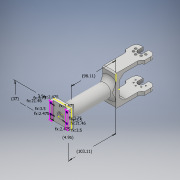
# Autodesk Inventor part: HuesitoJustina2
Saved by Autodesk Inventor 2018 (Build 220112000, 112)
## iProperties
Created: 2019-04-23
Part Number: HuesitoJustina2
Material: Genérico
Document SubType Name: Modeling
Designer: kille
Density: 1 g/cm^3
Appearance: Valor por defecto
Author: kille
Autodesk Inventor part; units mm, degrees
ref_plane "YZ Plane" through (0, 0, 0) normal (1, 0, 0) x (0, 1, 0)
ref_plane "XZ Plane" through (0, 0, 0) normal (0, 1, 0) x (-1, 0, 0)
ref_plane "XY Plane" through (0, 0, 0) normal (0, 0, 1) x (1, 0, 0)
sketch "Boceto1" plane through (0, 0, 0) normal (0, 1, 0) x (-1, 0, 0)
  line L0 (14.5, 26) -> (-14.5, 26)
  line L1 (-14.5, 26) -> (-14.5, -26)
  line L2 (-14.5, -26) -> (14.5, -26)
  line L3 (14.5, -26) -> (14.5, 26)
  point P0 (0, 0)
  dimension "d0" = 52
  dimension "d1" = 29
  dimension "d2" = 14.5
  dimension "d3" = 26
  constraints: 8 end point, 2 parallel, 1 horizontal, 1 perpendicular
  measures "d0" distance of L2.end L0.start
  measures "d1" distance of L0.start L0.end
  measures "d2" distance from line of point (0, 0) L3
  measures "d3" distance from line of point (0, 0) L0
extrude "Extrusión1" add sketch "Boceto1" against normal blind 7.5
sketch "Boceto2" plane through (-14.5, 0, 26) normal (0, 0, 1) x (1, 0, 0)
  line L0 (0, 0) -> (29, 0) projected
  line L1 (0, 0) -> (29, 0) projected
  line L2 (0, 0) -> (0, -7.5) projected
  line L3 (29, -7.5) -> (0, -7.5) projected
  line L4 (29, 0) -> (29, -7.5) projected
  line L5 (0, 0) -> (29, 0)
  line L6 (29, 0) -> (29, 67)
  line L7 (29, 67) -> (0, 67)
  line L8 (0, 67) -> (0, 0)
  point P0 (14.5, 0)
  dimension "d6" = 29
  dimension "d7" = 67
  dimension "d8" = 29
  constraints: 8 end point, 2 parallel, 1 horizontal, 1 perpendicular
  measures "d6" distance of L3.start L2.end
  measures "d7" distance of L5.end L6.end
  measures "d8" distance of L6.end L7.end
extrude "Extrusión2" add sketch "Boceto2" along normal blind 7.5 contours L8 L7 L6 L0
sketch "Boceto3" plane through (14.5, 0, -26) normal (0, 0, -1) x (-1, 0, 0)
  line L0 (29, 0) -> (0, 0) projected
  line L1 (29, 67) -> (29, 0) projected
  line L2 (0, 67) -> (29, 67) projected
  line L3 (0, 0) -> (0, 67) projected
  line L4 (0, 0) -> (29, 0) projected
  line L5 (0, 0) -> (0, -7.5) projected
  line L6 (29, -7.5) -> (0, -7.5) projected
  line L7 (29, 0) -> (29, -7.5) projected
  point P0 (14.5, 0)
extrude "Extrusión3" add sketch "Boceto3" along normal blind 7.5 contours L0 L3 L2 L1
sketch "Boceto4" plane through (14.5, -7.5, 26) normal (1, 0, 0) x (0, 0, -1)
  line L0 (52, 7.5) -> (52, 0) projected
  line L1 (52, 7.5) -> (59.5, 7.5) projected
  line L2 (0, 7.5) -> (-7.5, 7.5) projected
  line L3 (0, 7.5) -> (0, 0) projected
  line L4 (0, 7.5) -> (-7.5, 7.5)
  line L5 (-7.5, 7.5) -> (-7.5, 0)
  line L6 (-7.5, 0) -> (0, 0)
  line L7 (0, 0) -> (0, 7.5)
  line L8 (52, 7.5) -> (59.5, 7.5)
  line L9 (59.5, 7.5) -> (59.5, 0)
  line L10 (59.5, 0) -> (52, 0)
  line L11 (52, 0) -> (52, 7.5)
  point P0 (26, 7.5)
  dimension "d13" = 7.5
  dimension "d14" = 7.5
  dimension "d15" = 7.5
  dimension "d16" = 7.5
  constraints: 16 end point, 4 parallel, 2 horizontal, 2 perpendicular, 1 point on line
  measures "d13" distance of L8.end L9.end
  measures "d14" distance of L9.end L10.end
  measures "d15" distance of L4.end L5.end
  measures "d16" distance of L5.end L6.end
extrude "Extrusión4" add sketch "Boceto4" against normal blind 29
sketch "Boceto5" plane through (14.5, 0, 26) normal (1, 0, 0) x (0, 0, -1)
  line L0 (0, 0) -> (0, 67) projected
  line L1 (0, 0) -> (52, 0) projected
  line L2 (52, 67) -> (52, 0) projected
  line L3 (52, 0) -> (0, 0) projected
  line L4 (0, 10) -> (10, 0)
  line L5 (42, 0) -> (52, 10)
  point P0 (26, 0)
  dimension "d19" = 10
  dimension "d20" = 10
  dimension "d21" = 10
  dimension "d22" = 10
  constraints: 4 end point, 4 point on line
  measures "d19" distance of L0.start L4.start
  measures "d20" distance of L0.start L4.end
  measures "d21" distance of L1.end L5.start
  measures "d22" distance of L5.end L1.end
extrude "Extrusión5" add sketch "Boceto5" against normal blind 29
sketch "Boceto6" plane through (0, -7.5, 0) normal (0, -1, 0) x (1, 0, 0)
  circle A0 centre (0, 0) radius 14
  dimension "d26" = 28
  constraints: 1 centre point, 1 coincident
  measures "d26" diameter of A0
extrude "Extrusión6" add sketch "Boceto6" along normal blind 103.11
fillet "Empalme1" radius 10 1 edges at (-14, -7.5, 0)
fillet "Empalme2" radius 10 4 edges at (0, 10, -26) (0, 0, -16) (0, 0, 16) (0, 10, 26)
sketch "Boceto7" plane through (14.5, 0, -33.5) normal (0, 0, -1) x (-1, 0, 0)
  line L0 (29, 67) -> (29, -7.5) projected
  line L1 (29, 67) -> (0, 67) projected
  line L2 (0, 67) -> (0, -7.5) projected
  line L3 (0, -7.5) -> (29, -7.5) projected
  line L4 (29, 67) -> (0, 67) projected
  line L5 (19.5, 67) -> (9.5, 67)
  line L6 (9.5, 67) -> (9.5, 62)
  line L7 (9.5, 62) -> (19.5, 62)
  line L8 (19.5, 62) -> (19.5, 67)
  arc A0 (9.5, 62) -> (19.5, 62) centre (14.5, 62) ccw
  circle A1 centre (14.5, 50.85) radius 1.35
  circle A2 centre (25.65, 62) radius 1.35
  circle A3 centre (3.35, 62) radius 1.35
  circle A4 centre (22.6295, 54.3689) radius 1.35
  circle A5 centre (6.1262, 54.6378) radius 1.35
  point P0 (14.5, 0)
  point P1 (14.5, 67)
  dimension "d31" = 29
  dimension "d32" = 74.5
  dimension "d33" = 14.5
  dimension "d34" = 10
  dimension "d35" = 5
  dimension "d36" = 5
  dimension "d37" = 5
  dimension "d38" = 2.7
  dimension "d39" = 4.8
  dimension "d40" = 2.7
  dimension "d41" = 2.7
  dimension "d43" = 11.15
  dimension "d44" = 11.15
  dimension "d45" = 11.15
  dimension "d46" = 2.7
  dimension "d47" = 2.7
  dimension "d48" = 11.15
  dimension "d49" = 11.15
  constraints: 8 end point, 6 centre point, 2 parallel, 2 point on circle, 1 horizontal, 1 midpoint, 1 perpendicular, 1 point on line
  measures "d31" distance of L0.start L1.end
  measures "d32" distance of L0.start L0.end
  measures "d33" distance of point (14.5, 67) L0.start
  measures "d34" distance of L6.end L7.end
  measures "d35" distance of point (14.5, 67) L5.start
  measures "d36" distance of L7.end L5.start
  measures "d37" radius of A0
  measures "d38" diameter of A1
  measures "d40" diameter of A2
  measures "d41" diameter of A3
  measures "d43" distance of A1.centre A0.centre
  measures "d44" distance of A2.centre A0.centre
  measures "d45" distance of A0.centre A3.centre
  measures "d46" diameter of A4
  measures "d47" diameter of A5
  measures "d48" distance of A4.centre A0.centre
  measures "d49" distance of A5.centre A0.centre
extrude "Extrusión7" cut sketch "Boceto7" against normal blind 67 contours L8 L7 L6 L1 | A0 L7 | A1 | A2 | A3 | A4 | A5
sketch "Boceto8" plane through (0, -110.61, 0) normal (0, -1, 0) x (1, 0, 0)
  circle A0 centre (0, 0) radius 14 projected
  line L0 (20.125, 21.1) -> (-20.125, 21.1)
  line L1 (-20.125, 21.1) -> (-20.125, -19.15)
  line L2 (-20.125, -19.15) -> (20.125, -19.15)
  line L3 (20.125, -19.15) -> (20.125, 21.1)
  dimension "d52" = 40.25
  dimension "d53" = 40.25
  dimension "d55" = 28
  dimension "d89" = 20.125
  dimension "d90" = 21.1
  constraints: 8 end point, 2 parallel, 1 horizontal, 1 perpendicular
  measures "d52" distance of L2.end L0.start
  measures "d53" distance of L0.start L0.end
  measures "d55" diameter of A0
  measures "d89" distance from line of point (0, 0) L1
  measures "d90" distance from line of L0 point (0, 0)
extrude "Extrusión8" add sketch "Boceto8" along normal blind 4 contours A0 | L3 L2 L1 L0
sketch "Boceto14" plane through (-14.5, 0, 33.5) normal (0, 0, 1) x (1, 0, 0)
  circle A0 centre (3.35, 62) radius 1.35 projected
  circle A1 centre (6.3705, 54.3689) radius 1.35 projected
  circle A2 centre (14.5, 50.85) radius 1.35 projected
  circle A3 centre (22.8738, 54.6378) radius 1.35 projected
  circle A4 centre (25.65, 62) radius 1.35 projected
  circle A5 centre (3.35, 62) radius 2.4
  circle A6 centre (6.3705, 54.3689) radius 2.4
  circle A7 centre (14.5, 50.85) radius 2.4
  circle A8 centre (22.8738, 54.6378) radius 2.4
  circle A9 centre (25.65, 62) radius 2.4
  point P0 (14.5, 0)
  dimension "d91" = 4.8
  dimension "d92" = 4.8
  dimension "d93" = 4.8
  dimension "d94" = 4.8
  dimension "d95" = 4.8
  constraints: 5 centre point, 5 coincident
  measures "d91" diameter of A5
  measures "d92" diameter of A6
  measures "d93" diameter of A7
  measures "d94" diameter of A8
  measures "d95" diameter of A9
extrude "Extrusión14" cut sketch "Boceto14" against normal blind 5.5 contours A0 | A1 | A2 | A3 | A4 | A5 | A6 | A7 | A8 | A9
sketch "Boceto15" plane through (14.5, 0, -33.5) normal (0, 0, -1) x (-1, 0, 0)
  circle A0 centre (25.65, 62) radius 1.35 projected
  circle A1 centre (25.65, 62) radius 2.4 projected
  circle A2 centre (22.6295, 54.3689) radius 1.35 projected
  circle A3 centre (22.6295, 54.3689) radius 2.4 projected
  circle A4 centre (14.5, 50.85) radius 1.35 projected
  circle A5 centre (14.5, 50.85) radius 2.4 projected
  circle A6 centre (6.1262, 54.6378) radius 1.35 projected
  circle A7 centre (6.1262, 54.6378) radius 2.4 projected
  circle A8 centre (3.35, 62) radius 1.35 projected
  circle A9 centre (3.35, 62) radius 2.4 projected
  point P0 (14.5, 0)
extrude "Extrusión15" cut sketch "Boceto15" against normal blind 5.5 contours A0 | A1 | A2 | A3 | A4 | A5 | A6 | A7 | A8 | A9
sketch "Boceto16" plane through (0, -114.61, 0) normal (0, -1, 0) x (1, 0, 0)
  circle A0 centre (0, 0) radius 14 projected
  circle A1 centre (0, 0) radius 6.5
  dimension "d100" = 13
  constraints: 1 centre point, 1 coincident
  measures "d100" diameter of A1
extrude "Extrusión16" cut sketch "Boceto16" against normal blind 5 contours A1
sketch "Boceto17" plane through (0, -114.61, 0) normal (0, -1, 0) x (1, 0, 0)
  circle A0 centre (0, 0) radius 6.5 projected
  line L0 (20.125, 21.1) -> (-20.125, 21.1) projected
  line L1 (-20.125, 21.1) -> (-20.125, -19.15) projected
  line L2 (-20.125, -19.15) -> (20.125, -19.15) projected
  line L3 (20.125, -19.15) -> (20.125, 21.1) projected
  line L4 (-20.125, 21.1) -> (-20.125, -19.15) projected
  line L5 (-20.125, 21.1) -> (-15.175, 21.1)
  line L6 (-15.175, 21.1) -> (-15.175, -15.9)
  line L7 (-15.175, -15.9) -> (-20.125, -15.9)
  line L8 (-20.125, -15.9) -> (-20.125, 21.1)
  line L9 (20.125, 21.1) -> (15.175, 21.1)
  line L10 (15.175, 21.1) -> (15.175, -15.9)
  line L11 (15.175, -15.9) -> (20.125, -15.9)
  line L12 (20.125, -15.9) -> (20.125, 21.1)
  dimension "d103" = 37
  dimension "d104" = 4.95
  dimension "d105" = 37
  dimension "d106" = 4.95
  constraints: 16 end point, 4 parallel, 2 horizontal, 2 perpendicular
  measures "d103" distance of L5.end L6.end
  measures "d104" distance of L6.end L7.end
  measures "d105" distance of L9.end L10.end
  measures "d106" distance of L10.end L11.end
extrude "Extrusión17" add sketch "Boceto17" along normal blind 4 contours L3 L11 L10 L0 | L6 L7 L1 L0
sketch "Boceto18" plane through (-20.125, -110.61, -19.15) normal (-1, 0, 0) x (0, 0, 1)
  line L0 (40.25, 0) -> (0, 0) projected
  line L1 (0, 0) -> (0, -4) projected
  line L2 (3.25, -4) -> (0, -4) projected
  line L3 (3.25, -4) -> (3.25, -8) projected
  line L4 (40.25, -8) -> (3.25, -8) projected
  line L5 (40.25, 0) -> (40.25, -8) projected
  line L6 (0, 0) -> (0, -4) projected
  line L7 (0, 0) -> (3.25, -8)
  line L8 (3.25, -4) -> (3.25, -8) projected
  line L9 (3.25, -8) -> (3.25, -4)
  line L10 (3.25, -4) -> (1.625, -4)
  line L11 (0, -4) -> (3.25, -4) projected
  point P0 (19.15, 110.61)
  constraints: 6 end point, 2 midpoint, 1 collinear
extrude "Extrusión18" add sketch "Boceto18" against normal blind 4.95 contours L2 L3 L7
sketch "Boceto19" plane through (-20.125, -110.61, -19.15) normal (-1, 0, 0) x (0, 0, 1)
  line L0 (40.25, 0) -> (0, 0) projected
  line L1 (0, 0) -> (0, -4) projected
  line L2 (1.625, -4) -> (0, -4) projected
  line L3 (1.625, -4) -> (3.25, -8) projected
  line L4 (40.25, -8) -> (3.25, -8) projected
  line L5 (40.25, 0) -> (40.25, -8) projected
  line L6 (0, 0) -> (1.625, -4)
  line L7 (0, -4) -> (3.25, -4) projected
  line L8 (0, 0) -> (0, -4)
  line L9 (0, -4) -> (1.625, -4)
  point P0 (19.15, 110.61)
  constraints: 6 end point, 1 collinear, 1 perpendicular
extrude "Extrusión19" cut sketch "Boceto19" against normal blind 40.5 contours L6 L2 L1
sketch "Boceto20" plane through (20.125, -118.61, 21.1) normal (1, 0, 0) x (0, 0, -1)
  line L0 (38.625, 4) -> (40.25, 8) projected
  line L1 (40.25, 8) -> (0, 8) projected
  line L2 (0, 8) -> (0, 0) projected
  line L3 (37, 0) -> (0, 0) projected
  line L4 (37, 4) -> (37, 0) projected
  line L5 (38.625, 4) -> (37, 4) projected
  line L6 (37, 0) -> (38.625, 4) projected
  point P0 (21.1, 118.61)
extrude "Extrusión20" add sketch "Boceto20" against normal blind 4.95 contours L6 L4 L5
sketch "Boceto21" plane through (0, -118.61, 0) normal (0, -1, 0) x (1, 0, 0)
  line L0 (-20.125, 21.1) -> (-20.125, -15.9) projected
  line L1 (-20.125, -15.9) -> (-15.175, -15.9) projected
  line L2 (-15.175, -15.9) -> (-15.175, 21.1) projected
  line L3 (-15.175, 21.1) -> (-20.125, 21.1) projected
  line L4 (20.125, 21.1) -> (15.175, 21.1) projected
  line L5 (15.175, 21.1) -> (15.175, -15.9) projected
  line L6 (15.175, -15.9) -> (20.125, -15.9) projected
  line L7 (20.125, -15.9) -> (20.125, 21.1) projected
  circle A0 centre (-17.65, 17.35) radius 1.75
  circle A1 centre (-17.65, -4.11) radius 1.75
  circle A2 centre (17.65, 17.35) radius 1.75
  circle A3 centre (17.65, -4.11) radius 1.75
  line L8 (-20.125, 21.1) -> (-20.125, -15.9) projected
  line L9 (-20.125, -15.9) -> (-15.175, -15.9) projected
  line L10 (-15.175, -15.9) -> (-15.175, 21.1) projected
  line L11 (-15.175, 21.1) -> (-20.125, 21.1) projected
  line L12 (20.125, 21.1) -> (15.175, 21.1) projected
  line L13 (15.175, 21.1) -> (15.175, -15.9) projected
  line L14 (20.125, -15.9) -> (20.125, 21.1) projected
  line L15 (15.175, -15.9) -> (20.125, -15.9) projected
  point P0 (0, 0)
  dimension "d115" = 3.5
  dimension "d116" = 3.75
  dimension "d117" = 3.75
  dimension "d118" = 2.475
  dimension "d119" = 2.475
  dimension "d120" = 3.5
  dimension "d121" = 3.5
  dimension "d122" = 3.5
  dimension "d123" = 21.46
  dimension "d124" = 21.46
  dimension "d125" = 2.475
  dimension "d126" = 2.475
  dimension "d129" = 4.95
  dimension "d172" = 37
  constraints: 4 centre point
  measures "d115" diameter of A0
  measures "d116" distance from line of A0.centre L3
  measures "d117" distance from line of L4 A2.centre
  measures "d118" distance from line of L0 A0.centre
  measures "d119" distance from line of L7 A2.centre
  measures "d120" diameter of A2
  measures "d121" diameter of A1
  measures "d122" diameter of A3
  measures "d123" distance of A1.centre A0.centre
  measures "d124" distance of A2.centre A3.centre
  measures "d125" distance from line of L7 A3.centre
  measures "d126" distance from line of L0 A1.centre
  measures "d129" distance of L5.end L6.end
  measures "d172" distance of L0.start L0.end
sketch "Boceto22" plane through (0, -110.61, 0) normal (0, 1, 0) x (1, 0, 0)
  line L0 (20.125, -21.1) -> (-20.125, -21.1) projected
  line L1 (20.125, 19.15) -> (20.125, -21.1) projected
  line L2 (-20.125, 19.15) -> (20.125, 19.15) projected
  line L3 (-20.125, -21.1) -> (-20.125, 19.15) projected
  circle A0 centre (0, 0) radius 14 projected
sketch "Boceto23" plane through (-14.5, 0, 33.5) normal (0, 0, 1) x (1, 0, 0)
  circle A0 centre (22.8738, 54.6378) radius 2.4 projected
  circle A1 centre (6.3705, 54.3689) radius 2.4 projected
  circle A2 centre (3.35, 62) radius 2.4 projected
  circle A3 centre (14.5, 50.85) radius 2.4 projected
  circle A4 centre (25.65, 62) radius 2.4 projected
  line L0 (19.5, 67) -> (19.5, 62) projected
  arc A5 (9.5, 62) -> (19.5, 62) centre (14.5, 62) ccw projected
  line L1 (9.5, 62) -> (9.5, 67) projected
  line L2 (9.5, 67) -> (0, 67) projected
  line L3 (0, 67) -> (0, -7.5) projected
  line L4 (29, -7.5) -> (0, -7.5) projected
  line L5 (29, 67) -> (29, -7.5) projected
  line L6 (29, 67) -> (19.5, 67) projected
  line L7 (9.5, 67) -> (9.5, 62) projected
  line L8 (9.5, 67) -> (19.5, 67)
  line L9 (19.5, 67) -> (19.5, 62)
  line L10 (19.5, 62) -> (9.5, 62)
  line L11 (9.5, 62) -> (9.5, 67)
  line L12 (0, 67) -> (9.5, 67) projected
  arc A6 (9.5, 62) -> (19.5, 62) centre (14.5, 62) ccw projected
  line L13 (6.3705, 67) -> (9.5, 67)
  line L14 (9.5, 67) -> (9.5, 62)
  line L15 (9.5, 62) -> (6.3705, 62)
  line L16 (6.3705, 62) -> (6.3705, 67)
  line L17 (19.5, 67) -> (22.6295, 67)
  line L18 (22.6295, 67) -> (22.6295, 62)
  line L19 (22.6295, 62) -> (19.5, 62)
  line L20 (19.5, 62) -> (19.5, 67)
  line L21 (7.9352, 62) -> (7.9352, 67)
  line L22 (21.0648, 62) -> (21.0648, 67)
  line L23 (7.9352, 62) -> (9.5, 62)
  line L24 (9.5, 62) -> (9.5, 67)
  line L25 (9.5, 67) -> (7.9352, 67)
  line L26 (7.9352, 67) -> (7.9352, 62)
  line L27 (19.5, 62) -> (21.0648, 62)
  line L28 (21.0648, 62) -> (21.0648, 67)
  line L29 (21.0648, 67) -> (19.5, 67)
  line L30 (19.5, 67) -> (19.5, 62)
  line L31 (6.3705, 62) -> (7.9352, 62)
  line L32 (7.9352, 62) -> (7.9352, 67)
  line L33 (7.9352, 67) -> (6.3705, 67)
  line L34 (6.3705, 67) -> (6.3705, 62)
  line L35 (22.6295, 62) -> (21.0648, 62)
  line L36 (21.0648, 62) -> (21.0648, 67)
  line L37 (21.0648, 67) -> (22.6295, 67)
  line L38 (22.6295, 67) -> (22.6295, 62)
  arc A7 (6.3705, 62) -> (22.6295, 62) centre (14.5, 62) ccw
  point P0 (14.5, 0)
  dimension "d135" = 5
  dimension "d136" = 3.1295
  dimension "d137" = 3.1295
  constraints: 60 end point, 14 parallel, 7 horizontal, 7 perpendicular, 4 midpoint, 3 point on circle, 3 point on line, 1 centre point, 1 tangent
  measures "d135" distance of L15.end L13.start
  measures "d136" distance of L14.end L15.end
  measures "d137" distance of L18.end L19.end
extrude "Extrusión23" cut sketch "Boceto23" against normal blind 67 contours L6 L22 L19 L0 | L0 L10 L1 L8 | L19 A7 L15 A5 | A5 L10 | L6 L18 L19 L22 | L1 L15 L21 L2 | L21 L15 L16 L2
sketch "Boceto24" plane through (-14.5, 0, 33.5) normal (0, 0, 1) x (1, 0, 0)
  line L0 (22.6295, 67) -> (22.6295, 62) projected
  arc A0 (6.3705, 62) -> (22.6295, 62) centre (14.5, 62) ccw projected
  line L1 (6.3705, 62) -> (6.3705, 67) projected
  line L2 (6.3705, 67) -> (0, 67) projected
  line L3 (0, 67) -> (0, -7.5) projected
  line L4 (29, -7.5) -> (0, -7.5) projected
  line L5 (29, 67) -> (29, -7.5) projected
  line L6 (29, 67) -> (22.6295, 67) projected
  circle A1 centre (25.65, 62) radius 2.4 projected
  circle A2 centre (14.5, 50.85) radius 2.4 projected
  circle A3 centre (3.35, 62) radius 2.4 projected
  circle A4 centre (6.3705, 54.3689) radius 2.4 projected
  circle A5 centre (22.8738, 54.6378) radius 2.4 projected
  line L7 (0, 67) -> (6.3705, 67)
  line L8 (6.3705, 67) -> (6.3705, 73.3705)
  line L9 (6.3705, 73.3705) -> (0, 73.3705)
  line L10 (0, 73.3705) -> (0, 67)
  line L11 (29, 67) -> (22.6295, 67)
  line L12 (22.6295, 67) -> (22.6295, 73.3705)
  line L13 (22.6295, 73.3705) -> (29, 73.3705)
  line L14 (29, 73.3705) -> (29, 67)
  line L15 (0, 73.3705) -> (-6.3705, 73.3705)
  line L16 (-6.3705, 73.3705) -> (-6.3705, 49.3705)
  line L17 (-6.3705, 49.3705) -> (0, 49.3705)
  line L18 (0, 49.3705) -> (0, 73.3705)
  line L19 (29, 73.3705) -> (35.3705, 73.3705)
  line L20 (35.3705, 73.3705) -> (35.3705, 49.3705)
  line L21 (35.3705, 49.3705) -> (29, 49.3705)
  line L22 (29, 49.3705) -> (29, 73.3705)
  point P0 (14.5, 0)
  dimension "d141" = 6.3705
  dimension "d142" = 6.3705
  dimension "d143" = 6.3705
  dimension "d144" = 6.3705
  dimension "d145" = 6.3705
  dimension "d146" = 6.3705
  dimension "d147" = 6.3705
  dimension "d148" = 24
  dimension "d149" = 6.3705
  dimension "d150" = 24
  constraints: 32 end point, 8 parallel, 4 horizontal, 4 perpendicular, 1 point on line
  measures "d141" distance of L1.end L2.end
  measures "d142" distance of L5.start L0.start
  measures "d143" distance of L9.end L2.end
  measures "d144" distance of L8.end L9.end
  measures "d145" distance of L11.end L12.end
  measures "d146" distance of L12.end L13.end
  measures "d147" distance of L9.end L15.end
  measures "d148" distance of L15.end L16.end
  measures "d149" distance of L13.end L19.end
  measures "d150" distance of L19.end L20.end
extrude "Extrusión24" add sketch "Boceto24" against normal blind 7.5 contours L12 L13 L14 L6 | L14 L19 L20 L21 L5 | L2 L10 L9 L8 | L3 L17 L16 L15 L10
sketch "Boceto25" plane through (14.5, 0, -33.5) normal (0, 0, -1) x (-1, 0, 0)
  line L0 (6.3705, 62) -> (6.3705, 67) projected
  line L1 (6.3705, 67) -> (0, 67) projected
  line L2 (0, 67) -> (0, -7.5) projected
  line L3 (0, -7.5) -> (29, -7.5) projected
  line L4 (29, 67) -> (29, -7.5) projected
  line L5 (29, 67) -> (22.6295, 67) projected
  line L6 (22.6295, 67) -> (22.6295, 62) projected
  arc A0 (6.3705, 62) -> (22.6295, 62) centre (14.5, 62) ccw projected
  circle A1 centre (6.1262, 54.6378) radius 2.4 projected
  circle A2 centre (22.6295, 54.3689) radius 2.4 projected
  circle A3 centre (25.65, 62) radius 2.4 projected
  circle A4 centre (14.5, 50.85) radius 2.4 projected
  circle A5 centre (3.35, 62) radius 2.4 projected
  line L7 (6.3705, 62) -> (6.3705, 73.3705) projected
  line L8 (6.3705, 73.3705) -> (-6.3705, 73.3705) projected
  line L9 (-6.3705, 73.3705) -> (-6.3705, 49.3705) projected
  line L10 (-6.3705, 49.3705) -> (0, 49.3705) projected
  line L11 (0, 14.1421) -> (0, 49.3705) projected
  line L12 (29, 14.1421) -> (0, 14.1421) projected
  line L13 (29, 49.3705) -> (29, 14.1421) projected
  line L14 (29, 49.3705) -> (35.3705, 49.3705) projected
  line L15 (35.3705, 49.3705) -> (35.3705, 73.3705) projected
  line L16 (35.3705, 73.3705) -> (22.6295, 73.3705) projected
  line L17 (22.6295, 73.3705) -> (22.6295, 62) projected
  arc A6 (6.3705, 62) -> (22.6295, 62) centre (14.5, 62) ccw projected
  circle A7 centre (22.6295, 54.3689) radius 1.35 projected
  circle A8 centre (25.65, 62) radius 1.35 projected
  circle A9 centre (14.5, 50.85) radius 1.35 projected
  circle A10 centre (3.35, 62) radius 1.35 projected
  circle A11 centre (6.1262, 54.6378) radius 1.35 projected
  line L18 (35.3705, 49.3705) -> (35.3705, 73.3705) projected
  line L19 (35.3705, 49.3705) -> (29, 49.3705)
  line L20 (29, 49.3705) -> (29, 73.3705)
  line L21 (29, 73.3705) -> (35.3705, 73.3705)
  line L22 (35.3705, 73.3705) -> (35.3705, 49.3705)
  line L23 (35.3705, 73.3705) -> (22.6295, 73.3705) projected
  line L24 (22.6295, 73.3705) -> (29, 73.3705)
  line L25 (29, 73.3705) -> (29, 67)
  line L26 (29, 67) -> (22.6295, 67)
  line L27 (22.6295, 67) -> (22.6295, 73.3705)
  line L28 (6.3705, 73.3705) -> (0, 73.3705)
  line L29 (0, 73.3705) -> (0, 67)
  line L30 (0, 67) -> (6.3705, 67)
  line L31 (6.3705, 67) -> (6.3705, 73.3705)
  line L32 (-6.3705, 73.3705) -> (0, 73.3705)
  line L33 (0, 73.3705) -> (0, 49.3705)
  line L34 (0, 49.3705) -> (-6.3705, 49.3705)
  line L35 (-6.3705, 49.3705) -> (-6.3705, 73.3705)
  point P0 (14.5, 0)
  constraints: 32 end point, 8 parallel, 4 horizontal, 4 perpendicular, 1 midpoint
extrude "Extrusión25" add sketch "Boceto25" against normal blind 7.5 contours L1 L29 L8 L7 | L2 L10 L9 L8 L29 | L17 L16 L20 L5 | L20 L16 L15 L14 L4
fillet "Empalme7" radius 10 4 edges at (-14.5, 49.3705, -29.75) (-14.5, 49.3705, 29.75) (14.5, 49.3705, -29.75) (14.5, 49.3705, 29.75)
fillet "Empalme8" radius 10 4 edges at (-20.8705, 73.3705, 29.75) (-20.8705, 73.3705, -29.75) (20.8705, 73.3705, 29.75) (20.8705, 73.3705, -29.75)
sketch "Boceto26" plane through (0, -118.61, 0) normal (0, -1, 0) x (1, 0, 0)
  line L0 (-20.125, 21.1) -> (-20.125, -15.9) projected
  line L1 (-20.125, -15.9) -> (-15.175, -15.9) projected
  line L2 (-15.175, -15.9) -> (-15.175, 21.1) projected
  line L3 (-15.175, 21.1) -> (-20.125, 21.1) projected
  circle A0 centre (-17.65, 17.35) radius 1.75 projected
  circle A1 centre (-17.65, -4.11) radius 1.75 projected
  line L4 (20.125, 21.1) -> (15.175, 21.1) projected
  line L5 (15.175, 21.1) -> (15.175, -15.9) projected
  line L6 (15.175, -15.9) -> (20.125, -15.9) projected
  line L7 (20.125, -15.9) -> (20.125, 21.1) projected
  circle A2 centre (17.65, -4.11) radius 1.75 projected
  circle A3 centre (17.65, 17.35) radius 1.75 projected
  point P0 (0, 0)
extrude "Extrusión26" add sketch "Boceto22" along normal blind 5
fillet "Empalme9" radius 3 1 edges at (-14, -105.61, 0)
extrude "Extrusión27" cut sketch "Boceto26" against normal blind 13 contours A0 | A1 | A2 | A3
sketch "Boceto27" plane through (-14.5, 0, 33.5) normal (0, 0, 1) x (1, 0, 0)
  line L0 (6.3705, 62) -> (6.3705, 73.3705) projected
  line L1 (22.6295, 73.3705) -> (22.6295, 62) projected
  arc A0 (6.3705, 62) -> (22.6295, 62) centre (14.5, 62) ccw projected
  line L2 (6.3705, 73.3705) -> (8.3705, 73.3705)
  line L3 (8.3705, 73.3705) -> (8.3705, 62)
  line L4 (8.3705, 62) -> (6.3705, 62)
  line L5 (6.3705, 62) -> (6.3705, 73.3705)
  line L6 (22.6295, 73.3705) -> (20.6295, 73.3705)
  line L7 (20.6295, 73.3705) -> (20.6295, 62)
  line L8 (20.6295, 62) -> (22.6295, 62)
  line L9 (22.6295, 62) -> (22.6295, 73.3705)
  arc A1 (22.6295, 62) -> (22.6295, 62) centre (14.4992, 62) ccw
  line L10 (6.3705, 73.3705) -> (3.6295, 73.3705) projected
  line L11 (25.3705, 73.3705) -> (22.6295, 73.3705) projected
  arc A2 (8.3705, 62) -> (20.6295, 62) centre (14.5, 62) ccw
  arc A3 (6.3705, 62) -> (22.6295, 62) centre (14.5, 62) ccw
  line L12 (6.3705, 62) -> (8.3705, 62)
  line L13 (20.6295, 62) -> (22.6295, 62)
  point P0 (14.5, 0)
  dimension "d162" = 11.3705
  dimension "d163" = 11.3705
  dimension "d164" = 2
  dimension "d165" = 2
  dimension "d166" = 11.3705
  dimension "d167" = 11.3705
  constraints: 20 end point, 9 point on circle, 5 equal length, 3 centre point, 3 horizontal, 3 tangent, 2 perpendicular, 1 point on line, 1 other
  measures "d162" distance of L0.start L0.end
  measures "d163" distance of L1.start L1.end
  measures "d164" distance of L0.end L2.end
  measures "d165" distance of L1.start L6.end
  measures "d166" distance of L2.end L3.end
  measures "d167" distance of L6.end L7.end
extrude "Extrusión28" add sketch "Boceto27" against normal blind 7.5 contours L4 A2 L8 A0 | A1 L3 L4 | L0 L2 L3 A1 | A1 L7 L6 L1 | L8 L7 A1
sketch "Boceto28" plane through (14.5, 0, -33.5) normal (0, 0, -1) x (-1, 0, 0)
  arc A0 (8.3705, 62) -> (20.6295, 62) centre (14.5, 62) ccw projected
  arc A1 (6.3705, 62) -> (22.6295, 62) centre (14.5, 62) ccw projected
  line L0 (6.3705, 62) -> (6.3705, 73.3705) projected
  line L1 (8.3705, 62) -> (8.3705, 73.3705) projected
  line L2 (8.3705, 73.3705) -> (3.6295, 73.3705) projected
  line L3 (25.3705, 73.3705) -> (20.6295, 73.3705) projected
  line L4 (20.6295, 73.3705) -> (20.6295, 62) projected
  line L5 (22.6295, 73.3705) -> (22.6295, 62) projected
  point P0 (14.5, 0)
extrude "Extrusión29" add sketch "Boceto28" against normal blind 7.5
sketch "Boceto29" plane through (14.5, -7.5, 33.5) normal (1, 0, 0) x (0, 0, -1)
  line L0 (12.4, -98.11) -> (52.65, -98.11) projected
  line L1 (14.3754, 0) -> (0, 0) projected
  line L2 (52.65, -103.11) -> (12.4, -103.11) projected
  point P0 (33.5, 7.5)
  dimension "d173" = 98.11
  dimension "d174" = 103.11
  measures "d173" distance between parallel lines of L0 L1
  measures "d174" distance between parallel lines of L2 L1
fillet "Empalme10" radius 3 2 edges at (0, -7.5, 33.5) (0, -7.5, -33.5)
equation "\"d2\" = 0.5 * d1"
equation "\"d3\" = 0.5 * d0"
equation "\"d8\" = d6"
equation "\"d20\" = d19"
equation "\"d21\" = d20"
equation "\"d22\" = d21"
equation "\"d35\" = 0.5 * d34"
equation "\"d40\" = d38"
equation "\"d41\" = d38"
equation "\"d44\" = d43"
equation "\"d45\" = d44"
equation "\"d46\" = d38"
equation "\"d47\" = d38"
equation "\"d48\" = d45"
equation "\"d49\" = d48"
equation "\"d53\" = d52"
equation "\"d89\" = 0.5 * d53"
equation "\"d92\" = d91"
equation "\"d93\" = d92"
equation "\"d94\" = d93"
equation "\"d95\" = d92"
equation "\"d105\" = d103"
equation "\"d106\" = d104"
equation "\"d117\" = d116"
equation "\"d118\" = 0.5 * d129"
equation "\"d119\" = d118"
equation "\"d120\" = d115"
equation "\"d121\" = d115"
equation "\"d122\" = d120"
equation "\"d124\" = d123"
equation "\"d125\" = d118"
equation "\"d126\" = d118"
equation "\"d137\" = d136"
equation "\"d143\" = d141"
equation "\"d144\" = d141"
equation "\"d146\" = d142"
equation "\"d147\" = d144"
equation "\"d149\" = d147"
equation "\"d150\" = d148"
equation "\"d166\" = d162"
